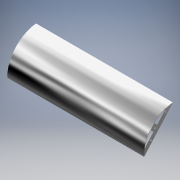
# Autodesk Inventor part: Kick Plate
Saved by Autodesk Inventor 2017 (Build 210142000, 142)
## iProperties
Created: 2017-01-14
Part Number: Kick Plate
Material: Generic
Document SubType Name: Modeling
Designer: Ben
Density: 1 g/cm^3
Appearance: Chrome - Polished
Author: Ben
Autodesk Inventor part; units mm, degrees
ref_plane "YZ Plane" through (0, 0, 0) normal (1, 0, 0) x (0, 1, 0)
ref_plane "XZ Plane" through (0, 0, 0) normal (0, 1, 0) x (-1, 0, 0)
ref_plane "XY Plane" through (0, 0, 0) normal (0, 0, 1) x (1, 0, 0)
sketch "Sketch1" plane through (0, 0, 0) normal (1, 0, 0) x (0, 1, 0)
  arc A0 (144.9614, 17.799) -> (0, 146.05) centre (0, 0) ccw
  line L0 (0, 0) -> (144.9614, 17.799) construction
  line L1 (0, 0) -> (0, 146.05) construction
  arc A1 (146.537, 17.9925) -> (0, 147.6375) centre (0, 0) ccw
  line L2 (0, 146.05) -> (0, 147.6375)
  line L3 (144.9614, 17.799) -> (146.537, 17.9925)
  dimension "d0" = 146.05
  dimension "d1" = 83
  dimension "d2" = 1.5875
  constraints: 8 end point, 4 point on circle, 2 centre point, 2 vertical, 1 coincident, 1 collinear
  measures "d0" radius of A0
  measures "d1" angle of L1 L0
  measures "d2" radial gap between concentric circles of A0 A1
extrude "Extrusion1" add sketch "Sketch1" along normal blind 612.775
sketch "Sketch2" plane through (612.775, 0, 0) normal (1, 0, 0) x (0, 0, -1)
  arc A0 (-17.799, 144.9614) -> (-146.05, 0) centre (0, 0) ccw construction
  line L0 (-146.05, 0) -> (0, 0) construction
  line L1 (-17.799, 144.9614) -> (0, 0) construction
  line L2 (0, 0) -> (-109.385, 96.7757) construction
  circle A1 centre (-97.8275, 86.5505) radius 3.175
  arc A2 (-17.9925, 146.537) -> (-147.6375, 0) centre (0, 0) ccw projected
  line L3 (-146.05, 0) -> (-17.799, 144.9614)
  line L4 (-47.9468, 139.635) -> (-87.7768, 94.6153)
  line L5 (-87.7768, 94.6153) -> (-101.7488, 106.9767)
  line L6 (-104.6074, 75.5919) -> (-118.5794, 87.9532)
  line L7 (-89.4123, 96.0622) -> (-106.2428, 77.0388) construction
  line L8 (-87.7768, 94.6153) -> (-104.6074, 75.5919) construction
  line L9 (-104.6074, 75.5919) -> (-144.4374, 30.5722)
  arc A3 (-101.7488, 106.9767) -> (-118.5794, 87.9532) centre (0, 0) ccw
  arc A4 (-144.4374, 30.5722) -> (-147.6375, 0) centre (0, 0) ccw
  line L10 (-147.6375, 0) -> (-146.05, 0) projected
  line L11 (-146.05, 0) -> (-147.6375, 0)
  arc A5 (-17.9925, 146.537) -> (-47.9468, 139.635) centre (0, 0) ccw
  line L12 (-17.799, 144.9614) -> (-17.9925, 146.537) projected
  line L13 (-17.9925, 146.537) -> (-17.799, 144.9614)
  line L14 (-54.9573, 131.7111) -> (-40.6897, 119.0882) construction
  circle A6 centre (-47.8235, 125.3997) radius 4.7625
  dimension "d5" = 6.35
  dimension "d6" = 130.6186
  dimension "d7" = 25.4
  dimension "d8" = 19.05
  dimension "d19" = 62.23
  dimension "d23" = 9.525
  constraints: 26 end point, 11 point on circle, 8 perpendicular, 6 point on line, 5 centre point, 3 coincident, 3 parallel, 2 midpoint, 1 horizontal
  measures "d5" diameter of A1
  measures "d6" distance of A1.centre point (0, 0)
  measures "d7" distance between parallel lines of L6 L5
  measures "d8" distance between parallel lines of L3 L4
  measures "d19" distance from line of L2 A6.centre
  measures "d23" diameter of A6
extrude "Extrusion2" add sketch "Sketch2" along normal blind 1.5875 contours L12 L3 L10 A2 L9 L6 L5 L4
sketch "Sketch3" plane through (0, 0, 0) normal (-1, 0, 0) x (0, 0, 1)
  arc A0 (146.05, 0) -> (142.2671, 33.0253) centre (0, 0) ccw projected
  line L0 (104.6074, 75.5919) -> (142.2671, 33.0253) projected
  line L1 (117.3859, 86.8973) -> (104.6074, 75.5919) projected
  arc A1 (117.3859, 86.8973) -> (100.5554, 105.9208) centre (0, 0) ccw projected
  line L2 (87.7768, 94.6153) -> (100.5554, 105.9208) projected
  line L3 (50.1171, 137.1819) -> (87.7768, 94.6153) projected
  arc A2 (50.1171, 137.1819) -> (17.799, 144.9614) centre (0, 0) ccw projected
  line L4 (146.05, 0) -> (17.799, 144.9614) projected
  circle A3 centre (97.8275, 86.5505) radius 3.175 projected
  arc A4 (146.05, 0) -> (17.799, 144.9614) centre (0, 0) ccw projected
  line L5 (146.05, 0) -> (147.6375, 0) projected
  arc A5 (147.6375, 0) -> (17.9925, 146.537) centre (0, 0) ccw projected
  line L6 (17.9925, 146.537) -> (17.799, 144.9614) projected
extrude "Extrusion3" add sketch "Sketch3" along normal blind 1.5875 contours L4 A2 L3 L2 A1 L1 L0 A0 | A0 A4 A1 A2 L6 A5 L5
body "Solid1"
